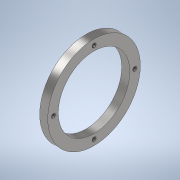
# Autodesk Inventor part: bear_89_140_in
Saved by Autodesk Inventor 2022.3 (Build 263350000, 350)
## iProperties
Created: 2022-06-17
Part Number: bear_89_140_in
Material: ステンレス鋼
Document SubType Name: Modeling
Designer: fhbdh
Density: 2.44666 g/cm^3
Appearance: 半つや出し
Mass: 100 g
Surface Area: 152.116 cm^2
Volume: 40.8721 cm^3
Author: fhbdh
Autodesk Inventor part; units mm, degrees
ref_plane "YZ Plane" through (0, 0, 0) normal (1, 0, 0) x (0, 1, 0)
ref_plane "XZ Plane" through (0, 0, 0) normal (0, 1, 0) x (-1, 0, 0)
ref_plane "XY Plane" through (0, 0, 0) normal (0, 0, 1) x (1, 0, 0)
sketch "スケッチ1" plane through (0, 0, 0) normal (1, 0, 0) x (0, 1, 0)
  circle A0 centre (0, 0) radius 44.5
  circle A1 centre (0, 0) radius 57.5
  dimension "d0" = 89
  dimension "d1" = 115
  constraints: 2 centre point, 2 coincident
  measures "d0" diameter of A0
  measures "d1" diameter of A1
extrude "押し出し1" add sketch "スケッチ1" along normal blind 10
sketch "スケッチ2" plane through (10, 0, 0) normal (1, 0, 0) x (0, 0, -1)
  point P0 (0, 0)
  point P1 (0, 50.5)
  point P2 (-50.5, 0)
  point P3 (0, -50.5)
  point P4 (50.5, 0)
  dimension "d4" = 50.5
  dimension "d7" = 360
  constraints: 5 other
  measures "d4" distance of point (0, 0) point (0, 50.5)
hole "穴1" at (10, 50.5, 0) at (10, 0, 50.5) at (10, -50.5, 0) at (10, 0, -50.5) direction (-1, 0, 0) diameter 5 end through all
